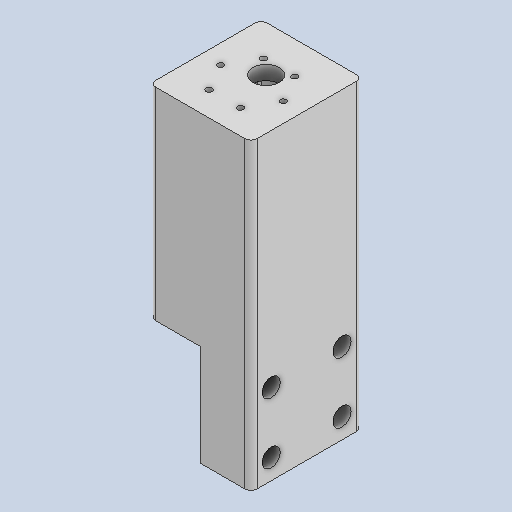
# Autodesk Inventor part: Link2_v2b
Saved by Autodesk Inventor 2022 (Build 260153000, 153)
## iProperties
Created: 2022-06-09
Part Number: Link2_v2b
Material: Generic
Document SubType Name: Modeling
Designer: Asus
Density: 1 g/cm^3
Appearance: Default
Author: Asus
Autodesk Inventor part; units mm, degrees
ref_plane "YZ Plane" through (0, 0, 0) normal (1, 0, 0) x (0, 1, 0)
ref_plane "XZ Plane" through (0, 0, 0) normal (0, 1, 0) x (-1, 0, 0)
ref_plane "XY Plane" through (0, 0, 0) normal (0, 0, 1) x (1, 0, 0)
sketch "Sketch1" plane through (0, 0, 0) normal (0, 1, 0) x (-1, 0, 0)
  line L0 (25, 32.5) -> (-25, 32.5)
  line L1 (-25, 32.5) -> (-25, -22.5)
  line L2 (-25, -22.5) -> (25, -22.5)
  line L3 (25, -22.5) -> (25, 32.5)
  circle A0 centre (0, 0) radius 15.2541
  dimension "d0" = 50
  dimension "d1" = 55
  dimension "d2" = 22.5
  dimension "d3" = 25
  constraints: 8 end point, 2 parallel, 1 centre point, 1 coincident, 1 horizontal, 1 perpendicular
  measures "d0" distance of L1.end L2.end
  measures "d1" distance of L0.end L1.end
  measures "d2" distance from line of point (0, 0) L2
  measures "d3" distance from line of point (0, 0) L3
extrude "Extrusion1" add sketch "Sketch1" along normal blind 150 contours L3 L2 L1 L0 | A0
sketch "Sketch2" plane through (0, 0, 0) normal (0, -1, 0) x (1, 0, 0)
  line L0 (-25, -22.5) -> (-25, 32.5) projected
  line L1 (-25, 32.5) -> (0, 32.5)
  line L2 (0, 32.5) -> (0, -22.5)
  line L3 (0, -22.5) -> (-25, -22.5)
  line L4 (-25, -22.5) -> (-25, 32.5)
  point P0 (0, 0)
  constraints: 8 end point, 2 parallel, 1 horizontal, 1 perpendicular
extrude "Extrusion2" cut sketch "Sketch2" against normal blind 50
sketch "Sketch3" plane through (0, 150, 0) normal (0, 1, 0) x (1, 0, 0)
  line L0 (-25, 22.5) -> (-25, -32.5) projected
  line L1 (25, -32.5) -> (25, 22.5) projected
  line L2 (-25, -32.5) -> (25, -32.5)
  line L3 (25, -32.5) -> (25, 22.5)
  line L4 (25, 22.5) -> (-25, 22.5)
  line L5 (-25, 22.5) -> (-25, -32.5)
  line L6 (-20, -27.5) -> (20, -27.5)
  line L7 (20, -27.5) -> (20, 17.5)
  line L8 (20, 17.5) -> (-20, 17.5)
  line L9 (-20, 17.5) -> (-20, -27.5)
  point P0 (0, 0)
  dimension "d8" = 5
  dimension "d9" = 5
  dimension "d10" = 5
  dimension "d11" = 5
  constraints: 16 end point, 4 parallel, 2 horizontal, 2 perpendicular
  measures "d8" distance between parallel lines of L4 L8
  measures "d9" distance between parallel lines of L0 L9
  measures "d10" distance between parallel lines of L2 L6
  measures "d11" distance between parallel lines of L1 L7
extrude "Extrusion3" cut sketch "Sketch3" against normal blind 100 contours L9 L8 L7 L6
fillet "Fillet1" radius 3 3 edges at (10, 50, -17.5) (20, 50, 5) (10, 50, 27.5)
sketch "Sketch4" plane through (0, 150, 0) normal (0, 1, 0) x (1, 0, 0)
  line L0 (25, -32.5) -> (25, 22.5) projected
  line L1 (-25, 22.5) -> (-25, -32.5) projected
  line L2 (25, -32.5) -> (-25, -32.5)
  line L3 (-25, -32.5) -> (-25, 22.5)
  line L4 (-25, 22.5) -> (25, 22.5)
  line L5 (25, 22.5) -> (25, -32.5)
  point P0 (0, 0)
  constraints: 8 end point, 2 parallel, 1 horizontal, 1 perpendicular
extrude "Extrusion4" add sketch "Sketch4" against normal blind 7
sketch "Sketch5" plane through (0, 150, 0) normal (0, 1, 0) x (1, 0, 0)
  circle A0 centre (0, 0) radius 6.5
  line L0 (0, -24.5) -> (0, 14.5) projected
  circle A1 centre (0, -7) radius 15.5
  line L1 (9.6514, -23.7167) -> (0, -7)
  line L2 (0, -7) -> (-9.5909, -23.612)
  line L3 (0, -7) -> (-18.6754, -7)
  line L4 (0, -7) -> (9.4872, 9.4324)
  line L5 (0, -7) -> (16.3511, -7)
  line L6 (0, -7) -> (-10.3523, 10.9308)
  circle A2 centre (15.5, -7) radius 1.5
  circle A3 centre (7.75, -20.4234) radius 1.5
  circle A4 centre (-7.75, -20.4234) radius 1.5
  circle A5 centre (-15.5, -7) radius 1.5
  circle A6 centre (-7.75, 6.4234) radius 1.5
  circle A7 centre (7.75, 6.4234) radius 1.5
  dimension "d17" = 31
  dimension "d18" = 7
  dimension "d19" = 13
  dimension "d20" = 60
  dimension "d21" = 60
  dimension "d22" = 60
  dimension "d23" = 60
  dimension "d24" = 60
  dimension "d25" = 30
  dimension "d26" = 3
  dimension "d27" = 3
  dimension "d28" = 3
  dimension "d29" = 3
  dimension "d30" = 3
  dimension "d31" = 3
  constraints: 12 end point, 8 centre point, 7 point on line, 6 point on circle, 1 coincident
  measures "d17" diameter of A1
  measures "d18" distance of L1.end point (0, 0)
  measures "d19" diameter of A0
  measures "d20" angle of L1 L2
  measures "d21" angle of L5 L1
  measures "d22" angle of L4 L5
  measures "d23" angle of L6 L4
  measures "d24" angle of L3 L2
  measures "d25" angle of L0 L6
  measures "d26" diameter of A2
  measures "d27" diameter of A7
  measures "d28" diameter of A6
  measures "d29" diameter of A5
  measures "d30" diameter of A4
  measures "d31" diameter of A3
extrude "Extrusion5" cut sketch "Sketch5" against normal blind 7 contours A0 L4 | L4 A0 L0 | L0 A0 L6 | A7 A1 L4 | L4 A1 A7 | L6 A0 | L4 A7 A1 | A1 A7 L4 | A3 A1 L1 | L1 A1 A3 | A4 A1 L2 | L2 A1 A4 | A5 A1 L3 | L3 A1 A5 | A2 A1 L5 | L5 A1 A2 | A6 A1 L6 | L6 A1 A6 | A1 L6 A6 | A2 A1 | A4 L2 A1 | A1 L1 A3 | A1 A3 L1 | L2 A4 A1 | L3 A5 A1 | A1 A5 L3 | A1 A6 L6 picked at (1.7263, 1.3919) picked at (-2.6431, 1.1884)
fillet "Fillet2" radius 3 2 edges at (0, 143, -17.5) (0, 143, 27.5)
fillet "Fillet3" radius 3 4 edges at (25, 75, 32.5) (25, 75, -22.5) (-25, 100, -22.5) (-25, 100, 32.5)
sketch "Sketch6" plane through (-25, 50, 29.5) normal (-1, 0, 0) x (0, 0, 1)
  line L0 (-2, 90) -> (-2, 0) projected
  line L1 (-47, 90) -> (-47, 3) projected
  line L2 (-2, 90) -> (-47, 90)
  line L3 (-47, 90) -> (-47, 10)
  line L4 (-47, 10) -> (-2, 10)
  line L5 (-2, 10) -> (-2, 90)
  line L6 (-49, 0) -> (0, 0) projected
  line L7 (-49, 100) -> (0, 100) projected
  line L8 (-4, 90) -> (-4, 10)
  line L9 (-45, 90) -> (-45, 10)
  line L10 (-52, 100) -> (-52, 0) projected
  point P0 (-29.5, -50)
  point P1 (3, 0)
  dimension "d36" = 10
  dimension "d38" = 10
  dimension "d39" = 7
  dimension "d40" = 7
  constraints: 12 end point, 6 point on line, 3 perpendicular, 2 parallel, 1 horizontal
  measures "d36" distance between parallel lines of L4 L6
  measures "d38" distance between parallel lines of L7 L2
  measures "d39" distance from line of point (3, 0) L8
  measures "d40" distance between parallel lines of L10 L9
extrude "Extrusion6" cut sketch "Sketch6" against normal blind 7 contours L8 L4 L9 L2
fillet "Fillet4" radius 3 4 edges at (-22.5, 140, 25.5) (-22.5, 60, 25.5) (-22.5, 60, -15.5) (-22.5, 140, -15.5)
sketch "Sketch7" plane through (0, 0, -22.5) normal (-1, 0, 0) x (0, 0, 1)
  line L0 (45, 40) -> (10, 40)
  line L1 (10, 40) -> (10, 10)
  line L2 (10, 10) -> (45, 10)
  line L3 (45, 10) -> (45, 40)
  line L4 (55, 50) -> (55, 0) projected
  line L5 (55, 0) -> (0, 0) projected
  line L6 (0, 0) -> (0, 50) projected
  line L7 (3, 50) -> (52, 50) projected
  circle A0 centre (45, 10) radius 1.95
  circle A1 centre (45, 40) radius 1.95
  circle A2 centre (10, 40) radius 1.95
  circle A3 centre (10, 10) radius 1.95
  point P0 (22.5, 0)
  dimension "d44" = 10
  dimension "d45" = 10
  dimension "d46" = 10
  dimension "d47" = 10
  dimension "d48" = 3.9
  dimension "d49" = 3.9
  dimension "d50" = 3.9
  dimension "d51" = 3.9
  constraints: 8 end point, 4 centre point, 4 coincident, 2 parallel, 1 horizontal, 1 perpendicular
  measures "d44" distance between parallel lines of L4 L3
  measures "d45" distance between parallel lines of L2 L5
  measures "d46" distance between parallel lines of L6 L1
  measures "d47" distance between parallel lines of L7 L0
  measures "d48" diameter of A0
  measures "d49" diameter of A1
  measures "d50" diameter of A2
  measures "d51" diameter of A3
extrude "Extrusion7" cut sketch "Sketch7" against normal blind 25 contours A2 L1 L0 | L0 L1 A2 | A1 L3 L0 | L0 L3 A1 | A3 L2 L1 | L1 L2 A3 | A0 L2 L3 | L3 L2 A0
sketch "Sketch8" plane through (25, 0, 29.5) normal (1, 0, 0) x (0, 0, -1)
  circle A0 centre (7, 10) radius 1.95 projected
  circle A1 centre (7, 10) radius 4.5
  circle A2 centre (7, 40) radius 1.95 projected
  circle A3 centre (7, 40) radius 4.5
  circle A4 centre (42, 40) radius 1.95 projected
  circle A5 centre (42, 40) radius 4.5
  circle A6 centre (42, 10) radius 1.95 projected
  circle A7 centre (42, 10) radius 4.5
  point P0 (29.5, 0)
  dimension "d54" = 9
  dimension "d55" = 9
  dimension "d56" = 9
  dimension "d57" = 9
  constraints: 4 centre point, 4 coincident
  measures "d54" diameter of A7
  measures "d55" diameter of A1
  measures "d56" diameter of A3
  measures "d57" diameter of A5
extrude "Extrusion8" cut sketch "Sketch8" against normal blind 10
body "Solid1"
